frameholder8000f120 (Autodesk Fusion 360 design; units mm, degrees)
Autodesk Fusion 360 part; units mm, degrees
sketch "Sketch1" plane through (0, 0, 0) normal (0, 0, 1) x (1, 0, 0)
  line L0 (-30.6, 30.8) -> (30.6, 30.8)
  line L1 (-30.6, 30.8) -> (-30.6, -69.6)
  line L2 (0, 30) -> (0, -70)
  line L3 (30.6, 30.8) -> (30.6, -69.6)
  line L4 (-30, 30.8) -> (-30, -70)
  line L5 (30, 30.8) -> (30, -70)
  line L6 (-30, 26.8) -> (30, 26.8)
  line L7 (-30, -66) -> (30, -66)
  line L8 (-33.5, 50) -> (-33.3333, 50)
  line L9 (33.3333, 50) -> (33.5, 50)
  line L10 (-30.6, -69.6) -> (30.6, -69.6)
  line L11 (-30.6, 30.8) -> (30.6, -69.6)
  line L12 (-30.6, -69.6) -> (30.6, 30.8)
  line L13 (40.6, -75.8) -> (-40.6, -75.8)
  line L14 (-40.6, -75.8) -> (-40.6, 35.8)
  line L15 (-40.6, 35.8) -> (40.6, 35.8)
  line L16 (40.6, 35.8) -> (40.6, -75.8)
  line L17 (40.6, -75.8) -> (-40.6, 35.8) construction
  line L18 (-40.6, -75.8) -> (40.6, 35.8) construction
  point P0 (-0.25, 0)
  point P1 (0, -20)
  dimension "d22" = 60
  dimension "d23" = 0.6
  dimension "d24" = 100.4
  dimension "d27" = 10
  dimension "d28" = 5
  constraint symmetric L0.start L2 L0.end
  constraint symmetric L1.end L2 L3.end
  constraint coincident L0 L4.start
  constraint symmetric L2 L4.start L5.start
  constraint symmetric L2 L4.end L5.end
  constraint coincident L4 L6.start
  constraint perpendicular L2 L6
  constraint coincident L4 L7.start
  constraint perpendicular L4 L7
  constraint collinear L8 L9
  constraint horizontal L13
  constraint perpendicular L13 L14
  constraint parallel L13 L15
  constraint parallel L14 L16
  constraint coincident L17 P1
  constraint coincident L18 P1
  constraint midpoint L2 P1
  measures "d22" distance of L4 L5
  measures "d23" distance of L1 L4
  measures "d24" distance of L0 L10
  measures "d27" distance of L1 L14
  measures "d28" distance of L0 L15
extrude "Extrude3" add sketch "Sketch1" along normal blind 2.8 contours L1 L4 L11 L12 | L0 L4 L11 | L0 L4 L5 L6 L11 L12 | L4 L10 L12 | L4 L6 L11 | L0 L5 L12 | L2 L4 L7 L10 L12 | L4 L7 L12 | L3 L5 L11 L12 | L5 L6 L12 | L2 L5 L7 L10 L11 | L5 L10 L11 | L5 L7 L11 makes body 1
extrude "Extrude4" add sketch "Sketch1" along normal blind 0.6 separate body makes body 2
fillet "Fillet3" radius 12.5 4 edges at (40.6, 35.8, 0.3) (40.6, -75.8, 0.3) (-40.6, -75.8, 0.3) (-40.6, 35.8, 0.3) on bodies 2
